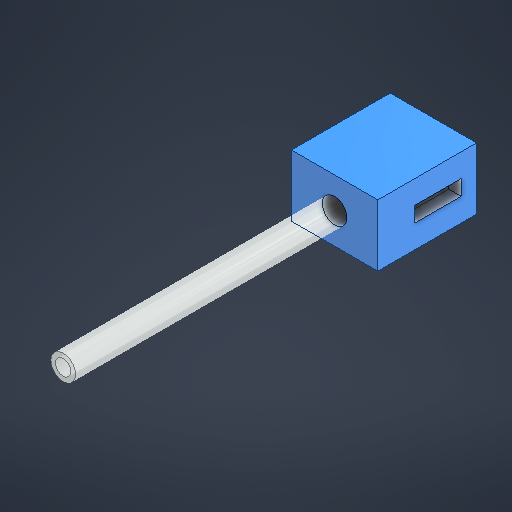
# Autodesk Inventor part: Деталь1
Saved by Autodesk Inventor 2025 (Build 290162010, 162A)
## iProperties
Created: 2024-11-10
Part Number: Деталь1
Material: Типовые
Document SubType Name: Modeling
Designer: Admin
Density: 1 g/cm^3
Appearance: По умолчанию
Author: Admin
Autodesk Inventor part; units mm, degrees
ref_plane "YZ Plane" through (0, 0, 0) normal (1, 0, 0) x (0, 1, 0)
ref_plane "XZ Plane" through (0, 0, 0) normal (0, 1, 0) x (-1, 0, 0)
ref_plane "XY Plane" through (0, 0, 0) normal (0, 0, 1) x (1, 0, 0)
sketch "Эскиз1" plane through (0, 0, 0) normal (0, 0, 1) x (1, 0, 0)
  circle A0 centre (0, 0) radius 2.5
  circle A1 centre (0, 0) radius 4
  dimension "d0" = 5
  dimension "d1" = 8
  constraints: 2 centre point, 2 coincident
  measures "d0" diameter of A0
  measures "d1" diameter of A1
extrude "Выдавливание1" add sketch "Эскиз1" along normal blind 100
sketch "Эскиз2" plane through (0, 0, 0) normal (0, 1, 0) x (-1, 0, 0)
  line L0 (4, 0) -> (-4, 0) projected
  line L1 (4, 0) -> (-4, 8)
  line L2 (-4, 0) -> (-4, 100) projected
  line L3 (4, 0) -> (4, 100) projected
  point P0 (0, 0)
  dimension "d4" = 45
  constraints: 2 end point, 1 point on line
  measures "d4" angle of L0 L1
extrude "Выдавливание2" cut sketch "Эскиз2" along normal through all both and the other way through all
sketch "Эскиз3" plane through (0, 0, 0) normal (0, 1, 0) x (-1, 0, 0)
  line L0 (-14, 12) -> (14, 12)
  line L1 (14, 12) -> (14, -20)
  line L2 (14, -20) -> (-14, -20)
  line L3 (-14, -20) -> (-14, 12)
  line L4 (-4, 8) -> (-4, 100) projected
  line L5 (4, 0) -> (4, 100) projected
  line L6 (-4, 8) -> (-14, 8)
  line L7 (4, 0) -> (-4, 8) projected
  line L8 (4, 0) -> (14, 0)
  line L9 (10, 8) -> (-10, 8)
  line L10 (-10, 8) -> (-10, -16)
  line L11 (-10, -16) -> (10, -16)
  line L12 (10, -16) -> (10, 8)
  line L13 (10, 0) -> (14, 0)
  line L14 (-10, 0) -> (-14, 0)
  line L15 (10, -15) -> (14, -15)
  line L16 (-10, -15) -> (-14, -15)
  point P0 (0, 0)
  dimension "d7" = 10
  dimension "d8" = 10
  dimension "d9" = 20
  dimension "d10" = 12
  dimension "d24" = 15
  constraints: 28 end point, 15 point on line, 5 perpendicular, 4 parallel, 1 collinear, 1 horizontal, 3 other
  measures "d7" distance between parallel lines of L1 L5
  measures "d8" distance between parallel lines of L4 L3
  measures "d9" distance from line of L2 L5.start
  measures "d10" distance from line of L0 L5.start
  measures "d24" distance between parallel lines of L13 L15
extrude "Выдавливание3" add sketch "Эскиз3" along normal mid plane 20 separate body
extrude "Выдавливание4" cut sketch "Эскиз3" along normal mid plane 5 contours L6 L10 L14 L3 | L7 L8 L12 L11 L10 L6 | L14 L10 L16 L3 | L16 L10 L11 L12 L15 L1 L2 L3 | L1 L15 L12 L8 bodies 2
combine bodies "Комбинировать1" operation type subtract main body 2 bodies to subtract 1 keep tools yes
extrude "Выдавливание5" cut sketch "Эскиз1" along normal through all both and the other way through all contours A0 bodies 2
sketch "Эскиз4" plane through (0, -10, 0) normal (0, -1, 0) x (1, 0, 0)
  line L0 (-14, -20) -> (14, -20) projected
  point P0 (0, 0)
sketch "Эскиз5" plane through (14, -10, 12) normal (1, 0, 0) x (0, 0, -1)
  line L0 (12, 7.5) -> (32, 7.5) projected
  line L1 (32, 7.5) -> (37, 7.5)
  line L2 (37, 7.5) -> (37, 5.5)
  line L3 (32, 0) -> (32, 7.5) projected
  line L4 (37, 5.5) -> (32, 0)
  line L5 (32, 10) -> (0, 10) projected
  line L6 (32, 12.5) -> (37, 12.5)
  line L7 (37, 12.5) -> (37, 14.5)
  line L8 (32, 20) -> (32, 12.5)
  line L9 (37, 14.5) -> (32, 20)
  point P0 (12, 10)
  dimension "d18" = 2
  dimension "d19" = 5
  constraints: 14 end point, 4 symmetric about line, 1 horizontal, 1 perpendicular
  measures "d18" distance of L1.end L2.end
  measures "d19" distance of L0.end L1.end
extrude "Выдавливание6" add sketch "Эскиз5" against normal up to surface (28 mm away) bodies 2
sketch "Эскиз6" plane through (0, 10, 0) normal (0, 1, 0) x (1, 0, 0)
  line L0 (14, 20) -> (-14, 20) projected
  line L1 (14, 25) -> (-14, 25) projected
  line L2 (-14, 20) -> (-4, 25)
  line L3 (14, 20) -> (4, 25)
  line L4 (-4, 0) -> (-4, -100) projected
  line L5 (4, -8) -> (4, -100) projected
  line L6 (14, 25) -> (14, 20) projected
  line L7 (-14, 25) -> (-14, 20) projected
  point P0 (0, 0)
  constraints: 4 end point, 2 point on line, 2 vertical alignment
extrude "Выдавливание7" cut sketch "Эскиз6" against normal through all contours L3 L1 L6 | L7 L1 L2 bodies 2
extrude "Выдавливание8" add sketch "Эскиз3" along normal mid plane 5 contours L6 L10 L14 L3 | L16 L10 L11 L12 L15 L1 L2 L3 bodies 2
sketch "Эскиз7" plane through (0, 2.5, 0) normal (0, -1, 0) x (1, 0, 0)
  line L0 (14, -20) -> (-14, -20) projected
  line L1 (-14, -20) -> (-4, -25) projected
  line L2 (4, -25) -> (-4, -25) projected
  line L3 (4, -25) -> (14, -20) projected
  point P0 (0, 0)
extrude "Выдавливание9" add sketch "Эскиз7" along normal blind 5 bodies 2
sketch "Эскиз8" plane through (0, 0, 0) normal (0, 1, 0) x (-1, 0, 0)
  line L0 (14, -15) -> (10, -15) projected
  line L1 (10, -15) -> (10, -16) projected
  line L2 (10, -16) -> (-10, -16) projected
  line L3 (-10, -16) -> (-10, -15) projected
  line L4 (-10, -15) -> (-14, -15) projected
  line L5 (-14, 0) -> (-14, -15) projected
  line L6 (-14, 0) -> (-10, 0) projected
  line L7 (-10, 0) -> (-10, 8) projected
  line L8 (-4, 8) -> (-10, 8) projected
  line L9 (-3.1225, 7.1225) -> (-4, 8) projected
  line L10 (3.1225, 0.8775) -> (-3.1225, 7.1225) projected
  line L11 (4, 0) -> (3.1225, 0.8775) projected
  line L12 (14, 0) -> (4, 0) projected
  line L13 (14, -15) -> (14, 0) projected
  line L14 (-4, -25) -> (4, -25) projected
  line L15 (10, -16) -> (4, -25)
  line L16 (-4, -25) -> (-10, -16)
  line L17 (10, -15) -> (10, 0)
  line L18 (-10, -15) -> (-10, 0)
  point P0 (0, 0)
  constraints: 8 end point, 1 parallel, 1 perpendicular, 1 point on line
extrude "Выдавливание10" cut sketch "Эскиз8" along normal mid plane 5 contours L15 L14 L16 L2 bodies 2
extrude "Выдавливание11" add sketch "Эскиз8" along normal mid plane 5 separate body contours L0 L17 L12 L13 | L4 L5 L6 L18
